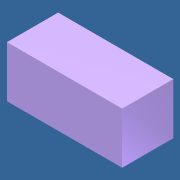
# Autodesk Inventor part: payload
Saved by Autodesk Inventor 2011 SP1 (Build 150282100, 282)
## iProperties
Created: 2010-12-21
Part Number: payload
Document SubType Name: Modeling
Designer: Antonella Wilby
Density: 0.5 g/cm^3
Material: Wood (Cherry)
Mass: 9438.95 g
Surface Area: 4541.93 cm^2
Volume: 18877.9 cm^3
Author: Antonella Wilby
Autodesk Inventor part; units mm, degrees
ref_plane "YZ Plane" through (0, 0, 0) normal (1, 0, 0) x (0, 1, 0)
ref_plane "XZ Plane" through (0, 0, 0) normal (0, 1, 0) x (-1, 0, 0)
ref_plane "XY Plane" through (0, 0, 0) normal (0, 0, 1) x (1, 0, 0)
sketch "Sketch1" plane through (0, 0, 0) normal (0, 0, 1) x (1, 0, 0)
  line L0 (-320.04, 0) -> (320.04, 0) projected
  line L1 (0, -142.24) -> (0, 142.24) projected
  line L2 (-228.6, 101.6) -> (228.6, 101.6)
  line L3 (228.6, 101.6) -> (228.6, -101.6)
  line L4 (228.6, -101.6) -> (-228.6, -101.6)
  line L5 (-228.6, -101.6) -> (-228.6, 101.6)
  point P0 (0, 0)
  point P1 (0, 101.6)
  point P2 (-228.6, 0)
  dimension "d0" = 203.2
  dimension "d1" = 457.2
  constraints: 8 end point, 2 midpoint, 2 parallel, 1 horizontal, 1 horizontal alignment, 1 perpendicular, 1 vertical alignment
  measures "d0" distance of L4.end L2.start
  measures "d1" distance of L2.start L2.end
extrude "Extrusion1" add sketch "Sketch1" along normal mid plane 203.2
body "Solid1"
